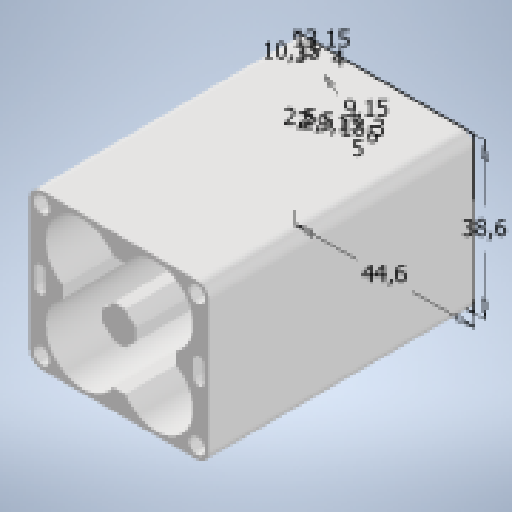
# Autodesk Inventor part: akkum
Saved by Autodesk Inventor 2025 (Build 290162000, 162)
## iProperties
Created: 2026-06-25
Part Number: akkum
Material: Типовые
Document SubType Name: Modeling
Designer: garin
Density: 1 g/cm^3
Appearance: По умолчанию
Author: garin
Autodesk Inventor part; units mm, degrees
ref_plane "YZ Plane" through (0, 0, 0) normal (1, 0, 0) x (0, 1, 0)
ref_plane "XZ Plane" through (0, 0, 0) normal (0, 1, 0) x (-1, 0, 0)
ref_plane "XY Plane" through (0, 0, 0) normal (0, 0, 1) x (1, 0, 0)
sketch "Эскиз1" plane through (0, 0, 0) normal (0, 0, 1) x (1, 0, 0)
  circle A0 centre (-9.15, 9.15) radius 9.15
  line L0 (0, 0) -> (-9.15, 0) construction
  line L1 (-9.15, 0) -> (-9.15, 9.15) construction
  line L2 (-9.15, 9.15) -> (0, 9.15) construction
  line L3 (0, 9.15) -> (0, 0) construction
  circle A1 centre (9.15, 9.15) radius 9.15
  circle A2 centre (-9.15, -9.15) radius 9.15
  circle A3 centre (9.15, -9.15) radius 9.15
  line L4 (0, 9.15) -> (-1.4869, 9.15) construction
  line L5 (-1.4869, 9.15) -> (-1.4869, 4.15) construction
  line L6 (-1.4869, 4.15) -> (0, 4.15) construction
  line L7 (0, 4.15) -> (0, 9.15) construction
  line L8 (-1.4869, 4.15) -> (1.4869, 4.15)
  line L9 (-1.4869, -4.15) -> (1.4869, -4.15)
  line L10 (-9.15, 0) -> (-4.15, 0) construction
  line L11 (-4.15, 0) -> (-4.15, 1.4869) construction
  line L12 (-4.15, 1.4869) -> (-9.15, 1.4869) construction
  line L13 (-9.15, 1.4869) -> (-9.15, 0) construction
  line L14 (-4.15, 1.4869) -> (-4.15, -1.4869)
  line L15 (4.15, 1.4869) -> (4.15, -1.4869)
  line L16 (-9.15, 9.15) -> (-22.3, 9.15) construction
  line L17 (-22.3, 9.15) -> (-22.3, 19.3) construction
  line L18 (-22.3, 19.3) -> (-9.15, 19.3) construction
  line L19 (-9.15, 19.3) -> (-9.15, 9.15) construction
  line L20 (-22.3, 19.3) -> (22.3, 19.3)
  line L21 (22.3, 19.3) -> (22.3, -19.3)
  line L22 (22.3, -19.3) -> (-22.3, -19.3)
  line L23 (-22.3, -19.3) -> (-22.3, 19.3)
  line L24 (-14.15, 1.4869) -> (-14.15, -1.4869)
  line L25 (-1.4869, 14.15) -> (1.4869, 14.15)
  line L26 (-1.4869, -14.15) -> (1.4869, -14.15)
  line L27 (14.15, 1.4869) -> (14.15, -1.4869)
  line L28 (-22.3, 19.3) -> (-19.3, 19.3) construction
  line L29 (-19.3, 19.3) -> (-19.3, 16.3) construction
  line L30 (-19.3, 16.3) -> (-22.3, 16.3) construction
  line L31 (-22.3, 16.3) -> (-22.3, 19.3) construction
  circle A4 centre (-19.3, 16.3) radius 2
  circle A5 centre (19.3, 16.3) radius 2
  circle A6 centre (-19.3, -16.3) radius 2
  circle A7 centre (19.3, -16.3) radius 2
  line L32 (-22.3, 0) -> (-19.8, 0) construction
  line L33 (-19.8, 0) -> (-19.8, 2) construction
  circle A8 centre (-19.8, 2) radius 1.25
  circle A9 centre (-19.8, -2) radius 1.25
  circle A10 centre (19.8, 2) radius 1.25
  circle A11 centre (19.8, -2) radius 1.25
  line L34 (-9.15, -9.15) -> (-22.3, -9.15) construction
  line L35 (-19.8, 2) -> (-21.05, 2) construction
  line L36 (-19.8, -2) -> (-21.05, -2) construction
  line L37 (-21.05, 2) -> (-21.05, -2)
  line L38 (-18.55, 2) -> (-18.55, -2)
  line L39 (21.05, 2) -> (21.05, -2)
  line L40 (18.55, 2) -> (18.55, -2)
  dimension "d22" = 2.5
  dimension "d0" = 18.3
  dimension "d1" = 9.15
  dimension "d2" = 9.15
  dimension "d3" = 5
  dimension "d4" = 5
  dimension "d5" = 13.15
  dimension "d6" = 10.15
  dimension "d7" = 44.6
  dimension "d8" = 38.6
  dimension "d17" = 3
  dimension "d18" = 3
  dimension "d19" = 4
  dimension "d20" = 2.5
  dimension "d21" = 2
  constraints: 82 end point, 27 symmetric about line, 12 parallel, 10 horizontal, 9 centre point, 9 perpendicular, 4 point on circle, 3 coincident, 2 point on line, 2 vertical, 1 midpoint, 1 tangent, 16 other
  measures "d0" diameter of A0
  measures "d1" distance of L1.end L2.end
  measures "d2" distance of L0.end L1.end
  measures "d3" distance of L5.end L4.end
  measures "d4" distance of L12.end L11.end
  measures "d5" distance of L17.end L18.end
  measures "d6" distance of L16.end L17.end
  measures "d7" distance of L21.end L22.end
  measures "d8" distance of L20.end L21.end
  measures "d17" distance of L29.end L30.end
  measures "d18" distance of L28.end L29.end
  measures "d19" diameter of A4
  measures "d20" distance of L32.start L32.end
  measures "d21" distance of L32.end L33.end
extrude "Выдавливание1" add sketch "Эскиз1" along normal blind 66 contours L8 A1 L15 A3 L9 A2 L14 A0 | L20 L21 L22 L23
fillet "Сопряжение1" radius 3 4 edges at (22.3, 19.3, 33) (22.3, -19.3, 33) (-22.3, 19.3, 33) (-22.3, -19.3, 33)
